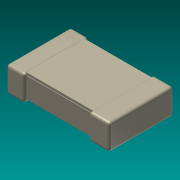
# Autodesk Inventor part: 0805 Resistor
Saved by Autodesk Inventor 2015 (Build 190159000, 159)
## iProperties
Created: 2014-10-16
Part Number: 0805 Resistor
Material: Generic
Document SubType Name: Modeling
Designer: Sawaiz Syed
Density: 1 g/cm^3
Appearance: Light Beige
Author: Sawaiz Syed
Autodesk Inventor part; units mm, degrees
ref_plane "YZ Plane" through (0, 0, 0) normal (1, 0, 0) x (0, 1, 0)
ref_plane "XZ Plane" through (0, 0, 0) normal (0, 1, 0) x (-1, 0, 0)
ref_plane "XY Plane" through (0, 0, 0) normal (0, 0, 1) x (1, 0, 0)
sketch "Sketch1" plane through (0, 0, 0) normal (0, 0, 1) x (1, 0, 0)
  line L0 (1, 0.625) -> (-1, 0.625)
  line L1 (-1, 0.625) -> (-1, -0.625)
  line L2 (-1, -0.625) -> (1, -0.625)
  line L3 (1, -0.625) -> (1, 0.625)
  line L4 (1, 0.625) -> (-1, -0.625) construction
  line L5 (-1, 0.625) -> (1, -0.625) construction
  point P0 (0, 0)
  dimension "d0" = 2
  dimension "d1" = 1.25
  constraints: 12 end point, 2 midpoint, 2 parallel, 1 horizontal, 1 perpendicular
  measures "d0" distance of L2.end L1.end
  measures "d1" distance of L1.end L0.end
extrude "Extrusion1" add sketch "Sketch1" along normal mid plane 0.5
sketch "Sketch2" plane through (0, 0, 0.25) normal (0, 0, 1) x (-1, 0, 0)
  line L0 (0.65, 0.6243) -> (0.65, -0.625)
  line L1 (-1, 0.625) -> (-0.6, 0.625)
  line L2 (-0.6, 0.625) -> (-0.6, -0.625)
  line L3 (-0.6, -0.625) -> (-1, -0.625)
  line L4 (-1, -0.625) -> (-1, 0.625)
  line L5 (-0.6, 0.625) -> (0.65, 0.625)
  line L6 (0.65, 0.625) -> (0.65, -0.625)
  line L7 (0.65, -0.625) -> (-0.6, -0.625)
  line L8 (-0.6, -0.625) -> (-0.6, 0.625)
  line L9 (1, -0.625) -> (1, 0.625) projected
  line L10 (-1, -0.625) -> (1, -0.625) projected
  line L11 (1, -0.625) -> (1, 0.625) projected
  line L12 (1, 0.625) -> (-1, 0.625) projected
  line L13 (-1, 0.625) -> (-1, -0.625) projected
  point P0 (0, 0)
  point P1 (0, -0.625)
  dimension "d5" = 0.4
  dimension "d11" = 0.35
  constraints: 18 end point, 4 parallel, 2 horizontal, 2 perpendicular, 1 midpoint, 1 point on line
  measures "d5" distance of L2.end L3.end
  measures "d11" distance between parallel lines of L9 L0
extrude "Extrusion2" cut sketch "Sketch2" against normal blind 0.05 contours L0 L7 L2 L5
mirror "Mirror1" about plane through (0, 0, 0) normal (0, 0, 1) of "Extrusion2"
sketch "Sketch3" plane through (1, -0.625, -0.25) normal (0, -1, 0) x (1, 0, 0)
  line L0 (-1.65, 0.45) -> (-0.4, 0.45)
  line L1 (-0.4, 0.45) -> (-0.4, 0.05)
  line L2 (-0.4, 0.05) -> (-1.65, 0.05)
  line L3 (-1.65, 0.05) -> (-1.65, 0.45)
  point P0 (-1, 0.25)
  constraints: 8 end point, 2 parallel, 1 horizontal, 1 perpendicular
extrude "Extrusion3" cut sketch "Sketch3" against normal blind 0.05
mirror "Mirror2" about plane through (0, 0, 0) normal (0, 1, 0) of "Extrusion3"
fillet "Fillet1" radius 0.05 24 edges at (0.8, 0.625, 0.25) (1, 0.625, 0) (0.8, 0.625, -0.25) (0.8, -0.625, -0.25) (1, -0.625, 0) (0.8, -0.625, 0.25) (-0.825, -0.625, 0.25) (-1, -0.625, 0) (-0.825, -0.625, -0.25) (1, 0, -0.25) (1, 0, 0.25) (-0.825, 0.625, 0.25) (-1, 0, 0.25) (-0.825, 0.625, -0.25) (-1, 0.625, 0) (-1, 0, -0.25) (-0.65, 0.625, 0) (-0.65, 0, 0.25) (-0.65, -0.625, 0) (-0.65, 0, -0.25) (0.6, 0.625, 0) (0.6, 0, -0.25) (0.6, -0.625, 0) (0.6, 0, 0.25)
sketch "Sketch4" plane through (0, 0, 0.2) normal (0, 0, 1) x (1, 0, 0)
  line L0 (0.6, 0.575) -> (-0.65, 0.575) projected
  line L1 (-0.65, -0.575) -> (-0.65, 0.575) projected
  line L2 (-0.65, -0.575) -> (0.6, -0.575) projected
  line L3 (0.6, 0.575) -> (0.6, -0.575) projected
  line L4 (-0.65, 0.575) -> (-0.7, 0.575) projected
  line L5 (-0.7, 0.575) -> (-0.7, -0.575) projected
  line L6 (-0.7, -0.575) -> (-0.65, -0.575) projected
  line L7 (-0.65, -0.575) -> (-0.65, 0.575) projected
  line L8 (0.6, -0.575) -> (0.65, -0.575) projected
  line L9 (0.65, -0.575) -> (0.65, 0.575) projected
  line L10 (0.65, 0.575) -> (0.6, 0.575) projected
  line L11 (0.6, 0.575) -> (0.6, -0.575) projected
  line L12 (-0.7, -0.575) -> (0.65, -0.575)
  line L13 (0.65, -0.575) -> (0.65, 0.575)
  line L14 (0.65, 0.575) -> (-0.7, 0.575)
  line L15 (-0.7, 0.575) -> (-0.7, -0.575)
  line L16 (-0.675, -0.565) -> (0.64, -0.565)
  line L17 (0.64, -0.565) -> (0.64, 0.565)
  line L18 (0.64, 0.565) -> (-0.675, 0.565)
  line L19 (-0.675, 0.565) -> (-0.675, -0.565)
  point P0 (0, 0)
  dimension "d12" = 0.01
  dimension "d13" = 0.01
  dimension "d14" = 0.01
  dimension "d15" = 0.025
  constraints: 16 end point, 4 parallel, 2 horizontal, 2 perpendicular
  measures "d12" distance between parallel lines of L0 L18
  measures "d13" distance between parallel lines of L2 L16
  measures "d14" distance between parallel lines of L9 L17
  measures "d15" distance between parallel lines of L5 L19
extrude "Extrusion4" add sketch "Sketch4" along normal blind 0.045 contours L18 L17 L16 L3 | L3 L16 L1 L18 | L1 L16 L19 L18
equation "\"d13\" = d12"
equation "\"d14\" = d13"
body "Solid1"
